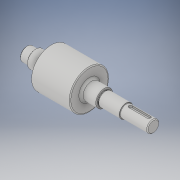
# Autodesk Inventor part: vratilo
Saved by Autodesk Inventor 2018 (Build 220112000, 112)
## iProperties
Created: 2018-05-05
Part Number: vratilo
Material: Generic
Document SubType Name: Modeling
Designer: Kristijan
Density: 1 g/cm^3
Appearance: Default
Author: Kristijan
Autodesk Inventor part; units mm, degrees
sketch "Sketch1" plane through (0, 0, 0) normal (1, 0, 0) x (0, 1, 0)
  circle A0 centre (0, 0) radius 36
  dimension "d0" = 72
  constraints: 1 centre point, 1 coincident
  measures "d0" diameter of A0
extrude "Extrusion1" add sketch "Sketch1" along normal mid plane 71
sketch "Sketch2" plane through (35.5, 0, 0) normal (1, 0, 0) x (0, 0, -1)
  circle A0 centre (0, 0) radius 15.5
  dimension "d3" = 31
  constraints: 1 centre point, 1 coincident
  measures "d3" diameter of A0
extrude "Extrusion2" add sketch "Sketch2" along normal blind 27
sketch "Sketch3" plane through (62.5, 0, 0) normal (1, 0, 0) x (0, 0, -1)
  circle A0 centre (0, 0) radius 12.5
  dimension "d6" = 25
  constraints: 1 centre point, 1 coincident
  measures "d6" diameter of A0
extrude "Extrusion3" add sketch "Sketch3" along normal blind 40
sketch "Sketch4" plane through (102.5, 0, 0) normal (1, 0, 0) x (0, 0, -1)
  circle A0 centre (0, 0) radius 11
  dimension "d9" = 22
  constraints: 1 centre point, 1 coincident
  measures "d9" diameter of A0
extrude "Extrusion4" add sketch "Sketch4" along normal blind 50
mirror "Mirror1" about plane through (0, 0, 0) normal (1, 0, 0) of "Extrusion2"
sketch "Sketch5" plane through (-62.5, 0, 0) normal (-1, 0, 0) x (0, 0, 1)
  circle A0 centre (0, 0) radius 12.5
  dimension "d12" = 25
  constraints: 1 centre point, 1 coincident
  measures "d12" diameter of A0
extrude "Extrusion5" add sketch "Sketch5" along normal blind 17
ref_plane "Work Plane1" through (102.5, 0, 11) normal (0, 0, 1) x (1, 0, 0)
sketch "Sketch6" plane through (102.5, 0, 11) normal (0, 0, 1) x (1, 0, 0)
  line L0 (8, 0) -> (42, 0) construction
  line L1 (8, -3) -> (42, -3)
  line L2 (42, 3) -> (8, 3)
  arc A0 (8, 3) -> (8, -3) centre (8, 0) ccw
  arc A1 (42, -3) -> (42, 3) centre (42, 0) ccw
  line L3 (50, -11) -> (50, 11) construction
  line L4 (-228.4, 0) -> (96.4, 0) construction
  line L5 (0, -12.5) -> (0, 12.5) construction
  point P0 (-102.5, 0)
  point P1 (25, 0)
  dimension "d15" = 34
  dimension "d16" = 6
  dimension "d18" = 5
  constraints: 8 end point, 4 point on circle, 4 tangent, 2 centre point, 1 collinear, 1 horizontal, 1 midpoint, 1 parallel
  measures "d15" distance of L0.start L0.end
  measures "d16" diameter of A1
  measures "d18" distance edge to line of A1 L3
extrude "Extrusion6" cut sketch "Sketch6" against normal blind 3.5
sketch "Sketch7" plane through (0, 0, 0) normal (0, 1, 0) x (-1, 0, 0)
  line L0 (-35.5, -15.5) -> (-62.5, -15.5) construction
  line L1 (-62.5, -15.5) -> (-62.5, -12.5) construction
  line L2 (-62.5, -12.5) -> (-102.5, -12.5) construction
  line L3 (-102.5, -12.5) -> (-102.5, -11) construction
  line L4 (-102.5, -11) -> (-152.5, -11) construction
  line L5 (-152.5, -11) -> (-152.5, 11) construction
  line L6 (-152.5, 11) -> (-147.5, 11) construction
  line L7 (-147.5, 11) -> (-147.5, 7.5) construction
  line L8 (-147.5, 7.5) -> (-107.5, 7.5) construction
  line L9 (-107.5, 7.5) -> (-107.5, 11) construction
  line L10 (-107.5, 11) -> (-102.5, 11) construction
  line L11 (-102.5, 11) -> (-102.5, 12.5) construction
  line L12 (-102.5, 12.5) -> (-62.5, 12.5) construction
  line L13 (-62.5, 12.5) -> (-62.5, 15.5) construction
  line L14 (-62.5, 15.5) -> (-35.5, 15.5) construction
  line L15 (-35.5, 15.5) -> (-35.5, 36) construction
  line L16 (-35.5, 36) -> (35.5, 36) construction
  line L17 (35.5, 36) -> (35.5, 15.5) construction
  line L18 (35.5, 15.5) -> (62.5, 15.5) construction
  line L19 (62.5, 15.5) -> (62.5, 12.5) construction
  line L20 (62.5, 12.5) -> (79.5, 12.5) construction
  line L21 (79.5, 12.5) -> (79.5, -12.5) construction
  line L22 (79.5, -12.5) -> (62.5, -12.5) construction
  line L23 (62.5, -12.5) -> (62.5, -15.5) construction
  line L24 (62.5, -15.5) -> (35.5, -15.5) construction
  line L25 (35.5, -15.5) -> (35.5, -36) construction
  line L26 (35.5, -36) -> (-35.5, -36) construction
  line L27 (-35.5, -36) -> (-35.5, -15.5) construction
  line L28 (-65, 15.4374) -> (-65, 12.5) construction
  line L29 (-62.5, 12.5) -> (-102.5, 12.5) construction
  line L30 (-65, 12.5) -> (-62.5, 12.5)
  line L31 (-62.5, 12.2) -> (-63.8804, 12.2)
  line L32 (-62.5, 15.5) -> (-62.5, -15.5) construction
  line L33 (-65, 12.5) -> (-63.8804, 12.2)
  line L34 (-62.5, 12.5) -> (-65, 12.5) construction
  line L35 (-62.5, 12.5) -> (-62.5, 12.2)
  line L36 (125.9, 0) -> (-198.9, 0) projected
  point P0 (0, 0)
  dimension "d21" = 2.5
  dimension "d24" = 0.3
  dimension "d25" = 15
  constraints: 12 end point, 3 point on line, 2 collinear, 2 horizontal, 1 vertical
  measures "d21" distance between parallel lines of L28 L13
  measures "d24" distance between parallel lines of L12 L31
  measures "d25" angle of L12 L33
revolve "Revolution1" cut sketch "Sketch7" angle 360 about axis through (-10, 0, 0) along (1, 0, 0)
mirror "Mirror2" about plane through (0, 0, 0) normal (1, 0, 0) of "Revolution1"
fillet "Fillet1" radius 0.6 1 edges at (62.5, 0, -12.2)
fillet "Fillet2" radius 0.6 1 edges at (63.8804, 0, -12.2)
fillet "Fillet3" radius 0.6 1 edges at (-62.5, 0, -12.2)
fillet "Fillet4" radius 0.6 1 edges at (-63.8804, 0, -12.2)
fillet "Fillet5" radius 0.6 1 edges at (102.5, 0, 11)
fillet "Fillet6" radius 4 2 edges at (35.5, 0, 15.5) (-35.5, 0, 15.5)
chamfer "Chamfer1" distance 1.5 angle 45 2 edges at (-79.5, 0, -12.5) (152.5, 0, 11)
chamfer "Chamfer2" distance 2 angle 30 1 edges at (35.5, -36, 0) measured on face at (35.5, -35.5, 0)
chamfer "Chamfer3" distance 2 angle 30 1 edges at (-35.5, -36, 0) measured on face at (-35.5, -35.5, 0)
body "Solid1"
